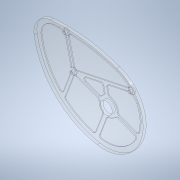
# Autodesk Inventor part: 足外フレーム
Saved by Autodesk Inventor 2022.2 (Build 262287010, 287A)
## iProperties
Created: 2022-01-10
Part Number: 足外フレーム
Material: Polycarbonate, Clear
Document SubType Name: Modeling
Designer: acps
Density: 1.2 g/cm^3
Appearance: Polycarbonate - Clear
Author: acps
Autodesk Inventor part; units mm, degrees
ref_plane "YZ Plane" through (0, 0, 0) normal (1, 0, 0) x (0, 1, 0)
ref_plane "XZ Plane" through (0, 0, 0) normal (0, 1, 0) x (-1, 0, 0)
ref_plane "XY Plane" through (0, 0, 0) normal (0, 0, 1) x (1, 0, 0)
sketch "Sketch1" plane through (0, 0, 0) normal (0, 0, 1) x (1, 0, 0)
  circle A0 centre (46.4683, 30) radius 14 construction
  circle A1 centre (66.4734, 20) radius 20.5 construction
  circle A2 centre (100, 0) radius 30 construction
  arc A3 (45.1112, 47.9488) -> (28.683, 27.2278) centre (46.4683, 30) ccw
  arc A4 (110.6259, 39.2116) -> (45.1112, 47.9488) centre (57.174, -111.5959) ccw
  arc A5 (91.0837, -36) -> (110.6259, 39.2116) centre (97.597, 2.4523) ccw
  arc A6 (28.683, 27.2278) -> (91.0837, -36) centre (103.7763, 38.9326) ccw
  line L0 (-13.9923, -60) -> (152.4896, -60) construction
  arc A7 (129.7918, 13.3835) -> (111.9633, 33.268) centre (97.597, 2.4523) ccw construction
  circle A8 centre (123.045, 25) radius 1.5
  circle A9 centre (100, 0) radius 3 construction
  arc A10 (93.5085, 39.0853) -> (53.6593, 43.3643) centre (57.174, -111.5959) ccw construction
  circle A11 centre (58.3063, 43.4) radius 1.5
  circle A12 centre (100, 0) radius 6.025
  circle A13 centre (65.359, 13) radius 1.5
  point P0 (0, 0)
  point P1 (0, 0)
  point P2 (78.3247, 47)
  dimension "d0" = 4
  dimension "d1" = 160
  dimension "d2" = 60
  dimension "d3" = 24
  dimension "d4" = 76
  dimension "d5" = 39
  dimension "d6" = 5
  dimension "d7" = 3
  dimension "d10" = 6
  dimension "d12" = 5
  dimension "d13" = 3
  dimension "d14" = 43.4
  dimension "d15" = 47
  dimension "d16" = 25
  dimension "d17" = 30
  dimension "d18" = 100
  dimension "d21" = 12.05
  dimension "d22" = 3
  dimension "d23" = 37
  dimension "d24" = 13
  constraints: 15 point on circle, 14 centre point, 4 tangent, 3 concentric, 2 coincident, 2 end point, 1 horizontal, 3 other
  measures "d0" radial gap between concentric circles of A0 A3
  measures "d1" radius of A4
  measures "d2" distance from line of L0 point (0, 0)
  measures "d3" distance from line of L0 A5.start
  measures "d4" radius of A6
  measures "d5" radius of A5
  measures "d6" radial gap between concentric circles of A5 A7
  measures "d7" diameter of A8
  measures "d10" diameter of A9
  measures "d12" radial gap between concentric circles of A4 A10
  measures "d13" diameter of A11
  measures "d14" vertical distance of point (0, 0) A11.centre
  measures "d15" vertical distance of point (0, 0) point (78.325, 47)
  measures "d16" vertical distance of point (0, 0) A8.centre
  measures "d17" vertical distance of point (0, 0) A3.centre
  measures "d18" distance of point (0, 0) point (100, 0)
  measures "d21" diameter of A12
  measures "d22" diameter of A13
  measures "d23" distance of A2.centre A13.centre
  measures "d24" vertical distance of point (0, 0) A13.centre
extrude "Extrusion1" add sketch "Sketch1" against normal blind 3
sketch "Sketch2" plane through (0, 0, -3) normal (0, 0, -1) x (-1, 0, 0)
  circle A0 centre (-123.045, 25) radius 3.01
  circle A1 centre (-58.3063, 43.4) radius 1.5 projected
  circle A2 centre (-58.3063, 43.4) radius 3.01
  circle A3 centre (-65.359, 13) radius 3.01
  point P0 (0, 0)
  point P1 (-100, 0)
  dimension "d25" = 6.02
  dimension "d26" = 6.02
  dimension "d27" = 6.02
  constraints: 3 centre point, 3 coincident
  measures "d25" diameter of A0
  measures "d26" diameter of A2
  measures "d27" diameter of A3
extrude "Extrusion2" cut sketch "Sketch2" against normal blind 1
sketch "Sketch4" plane through (0, 0, -3) normal (0, 0, -1) x (-1, 0, 0)
  circle A0 centre (100, 0) radius 28 construction
  line L0 (0, 0) -> (100, 0) construction
  circle A1 centre (100, 0) radius 30 construction
  circle A2 centre (66.4734, 20) radius 7 construction
  circle A3 centre (66.4734, 20) radius 9 construction
  circle A4 centre (66.4734, 20) radius 20 construction
  circle A5 centre (66.4734, 20) radius 20.5 construction
  circle A6 centre (46.4683, 30) radius 2 construction
  circle A7 centre (46.4683, 30) radius 2.5 construction
  circle A8 centre (46.4683, 30) radius 14 construction
  line L1 (0, 0) -> (0, 28) construction
  circle A9 centre (-66.4734, 20) radius 20.5 construction
  circle A10 centre (-46.4683, 30) radius 14 construction
  circle A11 centre (-100, 0) radius 30 construction
  circle A12 centre (-65.359, 13) radius 3.01 projected
  circle A13 centre (-58.3063, 43.4) radius 3.01 projected
  circle A14 centre (-123.045, 25) radius 3.01 projected
  arc A15 (-91.0837, -36) -> (-28.683, 27.2278) centre (-103.7763, 38.9326) ccw projected
  arc A16 (-28.683, 27.2278) -> (-45.1112, 47.9488) centre (-46.4683, 30) ccw projected
  arc A17 (-45.1112, 47.9488) -> (-110.6259, 39.2116) centre (-57.174, -111.5959) ccw projected
  arc A18 (-110.6259, 39.2116) -> (-91.0837, -36) centre (-97.597, 2.4523) ccw projected
  circle A19 centre (-100, 0) radius 6.025 projected
  arc A20 (-45.4882, 42.963) -> (-51.0229, 43.282) centre (-57.174, -111.5959) ccw
  arc A21 (-33.6234, 27.9979) -> (-45.4882, 42.963) centre (-46.4683, 30) ccw
  arc A22 (-91.9188, -31.0702) -> (-33.6234, 27.9979) centre (-103.7763, 38.9326) ccw
  arc A23 (-108.9556, 34.4989) -> (-120.1279, 27.9152) centre (-97.597, 2.4523) ccw
  circle A24 centre (-65.359, 13) radius 3.01 projected
  circle A25 centre (-65.359, 13) radius 3.01 projected
  arc A26 (-66.9207, 15.5732) -> (-66.0101, 16.831) centre (-67.9583, 17.2829) ccw
  arc A27 (-63.0877, 16.153) -> (-62.8239, 14.6227) centre (-61.1394, 15.701) ccw
  circle A28 centre (-58.3063, 43.4) radius 3.01 projected
  line L2 (-60.6419, 39.9702) -> (-66.0101, 16.831)
  line L3 (-63.0877, 16.153) -> (-58.0345, 37.9344)
  circle A29 centre (-65.359, 13) radius 1.5 projected
  line L4 (-58.3063, 43.4) -> (-65.359, 13) construction
  arc A30 (-60.6419, 39.9702) -> (-63.3814, 43.2798) centre (-63.2732, 40.5807) ccw
  circle A31 centre (-58.3063, 43.4) radius 3.01 projected
  arc A32 (-51.0229, 43.282) -> (-58.0345, 37.9344) centre (-51.2973, 36.3714) ccw
  arc A33 (-63.3814, 43.2798) -> (-108.9556, 34.4989) centre (-57.174, -111.5959) ccw
  arc A34 (-51.0229, 43.282) -> (-63.3814, 43.2798) centre (-57.174, -111.5959) ccw construction
  line L5 (-68.5631, 15.1986) -> (-119.5683, 25.8089)
  circle A35 centre (-123.045, 25) radius 1.5 projected
  line L6 (-123.045, 25) -> (-65.359, 13) construction
  arc A36 (-68.5631, 15.1986) -> (-67.0393, 15.4973) centre (-68.1557, 17.1567) ccw
  arc A37 (-120.1279, 27.9152) -> (-119.5683, 25.8089) centre (-119.3201, 27.0023) ccw
  arc A38 (-117.4108, 22.2958) -> (-128.4458, 16.7475) centre (-119.4337, 12.5714) ccw
  circle A39 centre (-123.045, 25) radius 3.01 projected
  arc A40 (-128.4458, 16.7475) -> (-91.9188, -31.0702) centre (-97.597, 2.4523) ccw
  arc A41 (-120.1279, 27.9152) -> (-128.4458, 16.7475) centre (-97.597, 2.4523) ccw construction
  arc A42 (-130.1287, -7.4315) -> (-127.5124, -8.7226) centre (-128.2151, -6.8501) ccw
  arc A43 (-126.1589, -11.419) -> (-127.1974, -14.2755) centre (-125.4562, -13.2915) ccw
  line L7 (-127.5124, -8.7226) -> (-110.3152, -2.2689)
  line L8 (-126.1589, -11.419) -> (-109.2611, -5.0776)
  line L9 (-100, 0) -> (-65.359, 13) construction
  arc A44 (-77.194, 10.1607) -> (-77.4894, 13.9913) centre (-77.8967, 12.0332) ccw
  line L10 (-77.4894, 13.9913) -> (-117.4108, 22.2958)
  circle A45 centre (-100, 0) radius 9.025
  line L11 (-108.8591, -1.7225) -> (-92.195, 4.5312) construction
  line L12 (-107.805, -4.5312) -> (-91.1409, 1.7225) construction
  line L13 (-92.195, 4.5312) -> (-90.7389, 5.0776) construction
  line L14 (-91.1409, 1.7225) -> (-89.6848, 2.2689) construction
  arc A46 (-92.9941, 5.6893) -> (-90.7389, 5.0776) centre (-91.4416, 6.9501) ccw
  arc A47 (-89.6848, 2.2689) -> (-90.9808, 0.3245) centre (-88.9821, 0.3964) ccw
  arc A48 (-107.0059, -5.6893) -> (-109.2611, -5.0776) centre (-108.5584, -6.9501) ccw
  arc A49 (-110.3152, -2.2689) -> (-109.0192, -0.3245) centre (-111.0179, -0.3964) ccw
  line L15 (-110.3152, -2.2689) -> (-108.8591, -1.7225) construction
  line L16 (-109.2611, -5.0776) -> (-107.805, -4.5312) construction
  line L17 (-89.6848, 2.2689) -> (-68.245, 10.3148)
  line L18 (-90.7389, 5.0776) -> (-77.194, 10.1607)
  arc A50 (-101.4929, 8.9007) -> (-99.8657, 10.4658) centre (-101.8238, 10.8731) ccw
  arc A51 (-95.9495, 9.6511) -> (-95.0814, 7.5669) centre (-93.9914, 9.2438) ccw
  arc A52 (-98.6419, 16.3487) -> (-100.1927, 18.7141) centre (-100.6, 16.756) ccw
  arc A53 (-92.3603, 17.0848) -> (-94.7258, 15.534) centre (-92.7677, 15.1267) ccw
  line L19 (-98.6419, 16.3487) -> (-99.8657, 10.4658)
  line L20 (-95.9495, 9.6511) -> (-94.7258, 15.534)
  line L21 (-100, 0) -> (-96.2765, 17.8994) construction
  arc A54 (-98.2628, -10.3215) -> (-100.1107, -9.0243) centre (-100.1353, -11.0242) ccw
  arc A55 (-93.9795, -6.7234) -> (-94.5178, -8.9161) centre (-92.6453, -8.2134) ccw
  arc A56 (-93.0239, -31.2388) -> (-91.4204, -28.5543) centre (-93.2929, -29.257) ccw
  arc A57 (-87.2536, -28.2728) -> (-84.848, -29.4978) centre (-85.3811, -27.5701) ccw
  line L22 (-98.2628, -10.3215) -> (-91.4204, -28.5543)
  line L23 (-94.5178, -8.9161) -> (-87.2536, -28.2728)
  line L24 (-100, 0) -> (-88.583, -30.4227) construction
  arc A58 (-57.8018, -15.1723) -> (-57.2244, -12.9455) centre (-59.0968, -13.6482) ccw
  arc A59 (-55.4567, -9.1173) -> (-52.1294, -9.787) centre (-53.5842, -8.4146) ccw
  line L25 (-57.2244, -12.9455) -> (-65.4825, 9.0599)
  line L26 (-55.4567, -9.1173) -> (-62.6951, 10.1709)
  line L27 (-65.359, 13) -> (-55.5396, -13.1656) construction
  arc A60 (-65.4825, 9.0599) -> (-68.245, 10.3148) centre (-67.4912, 8.3061) ccw
  arc A61 (-62.6336, 11.7224) -> (-62.6951, 10.1709) centre (-60.8226, 10.8736) ccw
  point P0 (-67.0393, 15.4973)
  point P1 (-62.8239, 14.6227)
  point P2 (-62.6336, 11.7224)
  dimension "d36" = 56
  dimension "d37" = 100
  dimension "d38" = 60
  dimension "d39" = 14
  dimension "d40" = 18
  dimension "d41" = 40
  dimension "d42" = 41
  dimension "d43" = 4
  dimension "d44" = 5
  dimension "d45" = 22.3653
  dimension "d46" = 28
  dimension "d47" = 39.0388
  dimension "d48" = 20
  dimension "d49" = 30
  dimension "d50" = 5
  dimension "d74" = 2
  dimension "d75" = 2
  dimension "d78" = 3
  dimension "d79" = 1.5
  dimension "d82" = 2
  dimension "d84" = 1.5
  dimension "d85" = 2
  dimension "d86" = 2
  dimension "d87" = 3
  dimension "d89" = 1.5
  dimension "d90" = 2
  dimension "d91" = 3
  dimension "d92" = 3
  dimension "d93" = 2
  dimension "d94" = 2
  dimension "d95" = 2
  dimension "d96" = 2
  dimension "d97" = 2
  dimension "d98" = 2
  dimension "d99" = 2
  dimension "d100" = 2
  dimension "d101" = 4
  dimension "d102" = 2
  dimension "d103" = 2
  dimension "d104" = 2
  dimension "d105" = 2
  dimension "d106" = 2
  dimension "d107" = 4
  dimension "d108" = 2
  dimension "d109" = 2
  dimension "d110" = 2
  dimension "d111" = 3
  dimension "d112" = 1.5
  dimension "d113" = 2
  constraints: 82 point on circle, 65 tangent, 56 end point, 46 centre point, 40 parallel, 7 coincident, 3 perpendicular, 3 point on line, 3 symmetric about line, 1 horizontal, 1 vertical, 30 other
  measures "d36" diameter of A0
  measures "d37" distance of A0.centre L0.start
  measures "d38" diameter of A1
  measures "d39" diameter of A2
  measures "d40" diameter of A3
  measures "d41" diameter of A4
  measures "d42" diameter of A5
  measures "d43" diameter of A6
  measures "d44" diameter of A7
  measures "d45" distance of A2.centre A6.centre
  measures "d46" diameter of A8
  measures "d47" distance of A0.centre A2.centre
  measures "d48" vertical distance of L0.start A2.centre
  measures "d49" vertical distance of L0.start A6.centre
  measures "d50" radial gap between concentric circles of A17 A20
  measures "d74" radius of A26
  measures "d75" radius of A27
  measures "d78" distance between parallel lines of L3 L2
  measures "d79" distance between parallel lines of L2 L4
  measures "d82" radius of A36
  measures "d84" distance between parallel lines of L5 L6
  measures "d85" radius of A42
  measures "d86" radius of A43
  measures "d87" distance between parallel lines of L8 L7
  measures "d89" distance between parallel lines of L7 L9
  measures "d90" radius of A44
  measures "d91" distance between parallel lines of L10 L5
  measures "d93" radius of A46
  measures "d94" radius of A47
  measures "d95" radius of A48
  measures "d96" radius of A49
  measures "d97" radius of A50
  measures "d98" radius of A51
  measures "d99" radius of A52
  measures "d100" radius of A53
  measures "d101" distance between parallel lines of L20 L19
  measures "d102" distance between parallel lines of L19 L21
  measures "d103" radius of A54
  measures "d104" radius of A55
  measures "d105" radius of A56
  measures "d106" radius of A57
  measures "d107" distance between parallel lines of L22 L23
  measures "d108" distance between parallel lines of L23 L24
  measures "d109" radius of A58
  measures "d110" radius of A59
  measures "d111" distance between parallel lines of L25 L26
  measures "d112" distance between parallel lines of L26 L27
  measures "d113" radius of A61
extrude "Extrusion3" cut sketch "Sketch4" against normal blind 1 contours A12 A27 L3 A32 A20 A21 A22 A59 L26 A61 | A12 A36 L5 A37 A23 A33 A30 L2 A26 | A60 L25 A58 A22 A57 L23 A55 A45 A47 L17 | A45 A51 L20 A53 L10 A44 L18 A46 | A38 L10 A52 L19 A50 A45 A49 L7 A42 A40 | A40 A43 L8 A48 A45 A54 L22 A56
equation "\"d79\" = 0.5 * d78"
body "Solid1"
